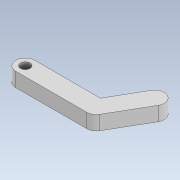
# Autodesk Inventor part: 夹爪01
Saved by Autodesk Inventor 2022.5 (Build 265521000, 521)
## iProperties
Created: 2024-11-12
Part Number: 夹爪01
Material: 常规
Document SubType Name: Modeling
Designer: Gagouking
Density: 1 g/cm^3
Appearance: 默认
Author: Gagouking
Autodesk Inventor part; units mm, degrees
ref_plane "YZ Plane" through (0, 0, 0) normal (1, 0, 0) x (0, 1, 0)
ref_plane "XZ Plane" through (0, 0, 0) normal (0, 1, 0) x (-1, 0, 0)
ref_plane "XY Plane" through (0, 0, 0) normal (0, 0, 1) x (1, 0, 0)
sketch "草图1" plane through (0, 0, 0) normal (0, 1, 0) x (-1, 0, 0)
  line L0 (0, 0) -> (-15, 0) construction
  line L1 (0, 2) -> (-15, 2)
  line L2 (-15, -2) -> (0, -2)
  arc A0 (0, -2) -> (0, 2) centre (0, 0) ccw
  arc A1 (-15, 2) -> (-15, -2) centre (-15, 0) ccw
  line L3 (-15, 0) -> (-19.5, -7.7942) construction
  line L4 (-13.2679, -1) -> (-17.7679, -8.7942)
  line L5 (-21.2321, -6.7942) -> (-16.7321, 1)
  arc A2 (-13.2679, -1) -> (-16.7321, 1) centre (-15, 0) ccw
  arc A3 (-21.2321, -6.7942) -> (-17.7679, -8.7942) centre (-19.5, -7.7942) ccw
  line L6 (-15, 0) -> (-6, 0) construction
  circle A4 centre (0, 0) radius 1
  point P0 (-7.5, 0)
  point P1 (-17.25, -3.8971)
  point P2 (-16.7321, 1)
  point P3 (-13.8453, -2)
  dimension "d0" = 15
  dimension "d1" = 2
  dimension "d2" = 9
  dimension "d3" = 120
  dimension "d4" = 2
  constraints: 18 end point, 9 tangent, 8 point on circle, 5 centre point, 2 horizontal, 2 midpoint, 2 parallel, 1 coincident, 1 equal length
  measures "d0" distance of L0.start L0.end
  measures "d1" radius of A1
  measures "d2" distance of L0.end L3.end
  measures "d3" angle of L3 L6
  measures "d4" diameter of A4
extrude "拉伸1" add sketch "草图1" along normal blind 3
